Autodesk Inventor part; units mm, degrees
(part 12 of 16)
  spline S72 degree 3 poles (40.8954, 83.9579) (41.0377, 83.8982) (41.1773, 83.832) (41.3128, 83.7584) (41.3531, 83.7365) (41.3931, 83.714) (41.4326, 83.6907) (41.4698, 83.6689) (41.5065, 83.6465) (41.5429, 83.6234) (41.577, 83.6018) (41.6107, 83.5797) (41.644, 83.557) (41.675, 83.5359) (41.7057, 83.5142) (41.7359, 83.4921) (41.764, 83.4715) (41.7917, 83.4506) (41.819, 83.4291) (41.8441, 83.4094) (41.869, 83.3892) (41.8934, 83.3686) (41.9158, 83.3499) (41.9378, 83.3307) (41.9595, 83.3112) (41.9791, 83.2935) (41.9984, 83.2755) (42.0175, 83.2572) (42.0346, 83.2409) (42.0515, 83.2243) (42.0677, 83.2072) (42.082, 83.1922) (42.0958, 83.1767) (42.1105, 83.1616) (42.138, 83.1336) (42.169, 83.1067) (42.1853, 83.0725) (42.1977, 83.0466) (42.2018, 83.0164) (42.2089, 82.9876) (42.2149, 82.9635) (42.223, 82.9404) (42.231, 82.9172) (42.2388, 82.8946) (42.2465, 82.8719) (42.2546, 82.8493) (42.2625, 82.8273) (42.2709, 82.8055) (42.2796, 82.7839) (42.288, 82.7627) (42.2968, 82.7417) (42.3059, 82.7209) (42.3148, 82.7005) (42.324, 82.6804) (42.3336, 82.6603) (42.3429, 82.6408) (42.3526, 82.6215) (42.3626, 82.6023) (42.3724, 82.5836) (42.3824, 82.565) (42.3929, 82.5467) (42.403, 82.5288) (42.4135, 82.511) (42.4244, 82.4935) (42.435, 82.4764) (42.4459, 82.4595) (42.4572, 82.4428) (42.4682, 82.4265) (42.4796, 82.4104) (42.4912, 82.3945) (42.5027, 82.379) (42.5145, 82.3637) (42.5266, 82.3487) (42.5385, 82.3339) (42.5508, 82.3194) (42.5634, 82.3052) (42.5758, 82.2912) (42.5885, 82.2776) (42.6016, 82.2642) (42.6145, 82.251) (42.6278, 82.2382) (42.6414, 82.2257) (42.6548, 82.2133) (42.6687, 82.2012) (42.6828, 82.1896) (42.697, 82.178) (42.7114, 82.1668) (42.7262, 82.1561) (42.7411, 82.1454) (42.7562, 82.1351) (42.7717, 82.1254) (42.7874, 82.1156) (42.8033, 82.1063) (42.8196, 82.0976) (42.8361, 82.0888) (42.853, 82.0806) (42.8701, 82.0731) (42.8876, 82.0654) (42.9055, 82.0584) (42.9236, 82.0522) (42.9421, 82.0459) (42.961, 82.0403) (42.9801, 82.0357) (42.9997, 82.0309) (43.0197, 82.027) (43.0397, 82.0242) (43.0604, 82.0212) (43.0813, 82.0194) (43.1023, 82.0187) (43.1239, 82.0179) (43.1456, 82.0184) (43.1672, 82.0201) (43.1894, 82.0219) (43.2116, 82.025) (43.2335, 82.0295) (43.2559, 82.034) (43.278, 82.04) (43.2996, 82.0472) (43.3151, 82.0524) (43.3303, 82.0581) (43.3454, 82.064) (43.4181, 82.0925) (43.4889, 82.1256) (43.5615, 82.1543) (43.6341, 82.183) (43.7084, 82.2072) (43.7809, 82.2361) (43.796, 82.2421) (43.811, 82.2484) (43.8258, 82.2552) (43.8465, 82.2647) (43.8668, 82.2754) (43.8862, 82.2874) (43.9053, 82.2991) (43.9235, 82.312) (43.941, 82.3259) (43.9579, 82.3394) (43.9741, 82.3539) (43.9894, 82.3692) (44.0041, 82.3841) (44.0181, 82.3997) (44.0313, 82.416) (44.044, 82.4318) (44.0559, 82.4482) (44.0669, 82.4652) (44.0777, 82.4816) (44.0877, 82.4985) (44.0969, 82.5159) (44.1058, 82.5328) (44.1141, 82.55) (44.1216, 82.5676) (44.129, 82.5848) (44.1357, 82.6023) (44.1417, 82.6201) (44.1476, 82.6375) (44.153, 82.6552) (44.1576, 82.6731) (44.1623, 82.6908) (44.1664, 82.7087) (44.1698, 82.7266) (44.1733, 82.7446) (44.1762, 82.7626) (44.1786, 82.7807) (44.181, 82.7989) (44.1829, 82.8171) (44.1843, 82.8354) (44.1857, 82.8538) (44.1865, 82.8722) (44.1869, 82.8907) (44.1874, 82.9094) (44.1873, 82.9281) (44.1868, 82.9467) (44.1863, 82.9657) (44.1853, 82.9847) (44.1839, 83.0036) (44.1825, 83.0228) (44.1807, 83.0421) (44.1784, 83.0612) (44.1761, 83.0808) (44.1734, 83.1003) (44.1703, 83.1198) (44.1671, 83.1396) (44.1635, 83.1595) (44.1595, 83.1792) (44.1555, 83.1994) (44.151, 83.2195) (44.1462, 83.2395) (44.1413, 83.2601) (44.1359, 83.2805) (44.1303, 83.3008) (44.1245, 83.3217) (44.1183, 83.3424) (44.1117, 83.363) (44.105, 83.3842) (44.098, 83.4052) (44.0906, 83.4261) (44.083, 83.4476) (44.075, 83.4689) (44.0668, 83.4901) (44.0583, 83.5119) (44.0495, 83.5335) (44.0402, 83.555) (44.0308, 83.577) (44.0208, 83.5988) (44.011, 83.6206) (44.001, 83.643) (43.9911, 83.6654) (43.979, 83.6871) (43.9646, 83.713) (43.9469, 83.7378) (43.9382, 83.7652) (43.9267, 83.8014) (43.931, 83.8421) (43.9318, 83.8814) (43.9323, 83.9025) (43.9318, 83.9231) (43.9319, 83.9439) (43.9321, 83.9675) (43.9331, 83.9911) (43.9344, 84.0148) (43.9359, 84.0411) (43.9376, 84.0675) (43.9399, 84.0938) (43.9423, 84.1229) (43.9453, 84.1519) (43.9488, 84.1809) (43.9526, 84.2126) (43.957, 84.2443) (43.9618, 84.2759) (43.9671, 84.3102) (43.973, 84.3445) (43.9794, 84.3786) (43.9863, 84.4155) (43.9939, 84.4523) (44.0021, 84.4889) (44.0109, 84.5282) (44.0203, 84.5674) (44.0305, 84.6064) (44.0412, 84.6481) (44.0528, 84.6897) (44.065, 84.731) (44.0779, 84.775) (44.0917, 84.8187) (44.1061, 84.8623) (44.1547, 85.0087) (44.2114, 85.1524) (44.2745, 85.2932) knots 0 0 0 0 0.065113 0.065113 0.065113 0.084473 0.084473 0.084473 0.102659 0.102659 0.102659 0.119672 0.119672 0.119672 0.135512 0.135512 0.135512 0.150178 0.150178 0.150178 0.163672 0.163672 0.163672 0.175991 0.175991 0.175991 0.187138 0.187138 0.187138 0.197111 0.197111 0.197111 0.205911 0.205911 0.205911 0.222284 0.222284 0.222284 0.234681 0.234681 0.234681 0.24506 0.24506 0.24506 0.255176 0.255176 0.255176 0.265035 0.265035 0.265035 0.274643 0.274643 0.274643 0.284008 0.284008 0.284008 0.293139 0.293139 0.293139 0.302047 0.302047 0.302047 0.310743 0.310743 0.310743 0.319241 0.319241 0.319241 0.327556 0.327556 0.327556 0.335706 0.335706 0.335706 0.343713 0.343713 0.343713 0.351599 0.351599 0.351599 0.359392 0.359392 0.359392 0.367126 0.367126 0.367126 0.374835 0.374835 0.374835 0.382562 0.382562 0.382562 0.390352 0.390352 0.390352 0.398256 0.398256 0.398256 0.406325 0.406325 0.406325 0.41461 0.41461 0.41461 0.423156 0.423156 0.423156 0.431994 0.431994 0.431994 0.441132 0.441132 0.441132 0.450548 0.450548 0.450548 0.460189 0.460189 0.460189 0.467051 0.467051 0.467051 0.5 0.5 0.5 0.532949 0.532949 0.532949 0.539811 0.539811 0.539811 0.549452 0.549452 0.549452 0.558868 0.558868 0.558868 0.568006 0.568006 0.568006 0.576844 0.576844 0.576844 0.58539 0.58539 0.58539 0.593675 0.593675 0.593675 0.601744 0.601744 0.601744 0.609648 0.609648 0.609648 0.617438 0.617438 0.617438 0.625165 0.625165 0.625165 0.632874 0.632874 0.632874 0.640608 0.640608 0.640608 0.648401 0.648401 0.648401 0.656287 0.656287 0.656287 0.664294 0.664294 0.664294 0.672444 0.672444 0.672444 0.680759 0.680759 0.680759 0.689257 0.689257 0.689257 0.697953 0.697953 0.697953 0.706861 0.706861 0.706861 0.715992 0.715992 0.715992 0.725357 0.725357 0.725357 0.734965 0.734965 0.734965 0.744824 0.744824 0.744824 0.75494 0.75494 0.75494 0.765319 0.765319 0.765319 0.777716 0.777716 0.777716 0.794089 0.794089 0.794089 0.802889 0.802889 0.802889 0.812862 0.812862 0.812862 0.824009 0.824009 0.824009 0.836328 0.836328 0.836328 0.849822 0.849822 0.849822 0.864488 0.864488 0.864488 0.880328 0.880328 0.880328 0.897341 0.897341 0.897341 0.915527 0.915527 0.915527 0.934887 0.934887 0.934887 1 1 1 1
  arc A275 (40.8954, 83.9579) -> (40.0961, 83.365) centre (45.7832, 76.5321) ccw
  spline S73 degree 3 poles (37.8374, 80.5191) (37.9904, 80.5386) (38.1444, 80.551) (38.2986, 80.5551) (38.3444, 80.5563) (38.3903, 80.5567) (38.4362, 80.5564) (38.4793, 80.556) (38.5223, 80.555) (38.5654, 80.5532) (38.6057, 80.5516) (38.6459, 80.5493) (38.6861, 80.5462) (38.7235, 80.5434) (38.7609, 80.54) (38.7982, 80.536) (38.8327, 80.5322) (38.8672, 80.5279) (38.9016, 80.523) (38.9333, 80.5184) (38.9648, 80.5134) (38.9963, 80.5078) (39.0251, 80.5027) (39.0537, 80.4972) (39.0823, 80.4911) (39.1081, 80.4856) (39.1338, 80.4796) (39.1595, 80.4734) (39.1824, 80.4677) (39.2054, 80.4619) (39.228, 80.4552) (39.2479, 80.4493) (39.2675, 80.4428) (39.2878, 80.4371) (39.3257, 80.4265) (39.3659, 80.4188) (39.3972, 80.3973) (39.4209, 80.3811) (39.4395, 80.3569) (39.4601, 80.3356) (39.4773, 80.3177) (39.4959, 80.3018) (39.5144, 80.2857) (39.5324, 80.27) (39.5504, 80.2541) (39.5687, 80.2386) (39.5866, 80.2236) (39.6047, 80.2089) (39.6231, 80.1945) (39.641, 80.1804) (39.6591, 80.1666) (39.6774, 80.1531) (39.6953, 80.1399) (39.7134, 80.1271) (39.7317, 80.1145) (39.7495, 80.1023) (39.7676, 80.0903) (39.7858, 80.0787) (39.8036, 80.0674) (39.8216, 80.0564) (39.8398, 80.0457) (39.8576, 80.0353) (39.8756, 80.0252) (39.8937, 80.0154) (39.9114, 80.0059) (39.9294, 79.9967) (39.9475, 79.9879) (39.9652, 79.9793) (39.9831, 79.971) (40.0011, 79.9631) (40.0188, 79.9554) (40.0367, 79.948) (40.0547, 79.9411) (40.0724, 79.9343) (40.0902, 79.9278) (40.1082, 79.9219) (40.1259, 79.9159) (40.1438, 79.9105) (40.1618, 79.9054) (40.1796, 79.9005) (40.1975, 79.896) (40.2155, 79.8919) (40.2334, 79.8879) (40.2514, 79.8844) (40.2695, 79.8815) (40.2875, 79.8785) (40.3056, 79.876) (40.3238, 79.8742) (40.342, 79.8723) (40.3603, 79.871) (40.3786, 79.8703) (40.397, 79.8696) (40.4155, 79.8696) (40.4339, 79.8702) (40.4526, 79.8708) (40.4713, 79.8721) (40.49, 79.8742) (40.509, 79.8763) (40.5279, 79.8792) (40.5466, 79.8828) (40.5659, 79.8866) (40.585, 79.8912) (40.6039, 79.8968) (40.6233, 79.9024) (40.6425, 79.9091) (40.6612, 79.9166) (40.6807, 79.9245) (40.6997, 79.9333) (40.7182, 79.9431) (40.7373, 79.9533) (40.7558, 79.9646) (40.7737, 79.9769) (40.7921, 79.9895) (40.8097, 80.0033) (40.8264, 80.0181) (40.8435, 80.0332) (40.8596, 80.0495) (40.8748, 80.0666) (40.8856, 80.0787) (40.8959, 80.0913) (40.9061, 80.104) (40.9548, 80.165) (40.9996, 80.2291) (41.0481, 80.2902) (41.0966, 80.3513) (41.1489, 80.4094) (41.1972, 80.4708) (41.2072, 80.4835) (41.2171, 80.4964) (41.2265, 80.5097) (41.2397, 80.5284) (41.2519, 80.5478) (41.2628, 80.5679) (41.2734, 80.5875) (41.2828, 80.6078) (41.2909, 80.6286) (41.2988, 80.6487) (41.3056, 80.6694) (41.3111, 80.6903) (41.3165, 80.7105) (41.3208, 80.7311) (41.324, 80.7517) (41.3271, 80.7718) (41.3292, 80.7919) (41.3304, 80.8122) (41.3315, 80.8318) (41.3316, 80.8514) (41.3309, 80.871) (41.3303, 80.8901) (41.3288, 80.9092) (41.3265, 80.9282) (41.3243, 80.9468) (41.3213, 80.9653) (41.3177, 80.9837) (41.3141, 81.0018) (41.3098, 81.0198) (41.305, 81.0376) (41.3001, 81.0552) (41.2947, 81.0727) (41.2888, 81.09) (41.2828, 81.1073) (41.2763, 81.1244) (41.2693, 81.1413) (41.2623, 81.1582) (41.2548, 81.1749) (41.2469, 81.1914) (41.2389, 81.2081) (41.2304, 81.2245) (41.2215, 81.2407) (41.2125, 81.2571) (41.2031, 81.2732) (41.1934, 81.2891) (41.1834, 81.3053) (41.1731, 81.3212) (41.1625, 81.3369) (41.1516, 81.3529) (41.1404, 81.3686) (41.1289, 81.3841) (41.1171, 81.3999) (41.105, 81.4154) (41.0925, 81.4307) (41.0798, 81.4463) (41.0668, 81.4617) (41.0535, 81.4768) (41.0399, 81.4923) (41.026, 81.5075) (41.0118, 81.5224) (40.9973, 81.5377) (40.9825, 81.5527) (40.9674, 81.5675) (40.9519, 81.5826) (40.9362, 81.5975) (40.9202, 81.6121) (40.9039, 81.6271) (40.8872, 81.6418) (40.8704, 81.6562) (40.8531, 81.671) (40.8355, 81.6854) (40.8177, 81.6997) (40.7995, 81.7143) (40.7811, 81.7286) (40.7623, 81.7426) (40.7431, 81.7569) (40.7236, 81.7708) (40.7042, 81.7849) (40.6843, 81.7992) (40.6646, 81.8137) (40.6432, 81.8264) (40.6178, 81.8416) (40.5901, 81.8542) (40.5689, 81.8736) (40.5408, 81.8993) (40.5242, 81.9367) (40.5053, 81.9711) (40.4951, 81.9896) (40.4843, 82.0072) (40.4741, 82.0253) (40.4625, 82.0458) (40.4515, 82.0668) (40.4408, 82.0879) (40.4289, 82.1115) (40.4172, 82.1351) (40.406, 82.159) (40.3936, 82.1854) (40.3817, 82.2121) (40.3702, 82.2389) (40.3576, 82.2683) (40.3456, 82.2979) (40.334, 82.3277) (40.3214, 82.3601) (40.3093, 82.3927) (40.2978, 82.4255) (40.2854, 82.4609) (40.2736, 82.4965) (40.2624, 82.5323) (40.2503, 82.5708) (40.2389, 82.6094) (40.2281, 82.6483) (40.2166, 82.6898) (40.2059, 82.7315) (40.1957, 82.7734) (40.185, 82.818) (40.175, 82.8628) (40.1658, 82.9077) (40.1347, 83.0588) (40.1118, 83.2116) (40.0961, 83.365) knots 0 0 0 0 0.065113 0.065113 0.065113 0.084473 0.084473 0.084473 0.102659 0.102659 0.102659 0.119672 0.119672 0.119672 0.135512 0.135512 0.135512 0.150178 0.150178 0.150178 0.163672 0.163672 0.163672 0.175991 0.175991 0.175991 0.187138 0.187138 0.187138 0.197111 0.197111 0.197111 0.205911 0.205911 0.205911 0.222284 0.222284 0.222284 0.234681 0.234681 0.234681 0.24506 0.24506 0.24506 0.255176 0.255176 0.255176 0.265035 0.265035 0.265035 0.274643 0.274643 0.274643 0.284008 0.284008 0.284008 0.293139 0.293139 0.293139 0.302047 0.302047 0.302047 0.310743 0.310743 0.310743 0.319241 0.319241 0.319241 0.327556 0.327556 0.327556 0.335706 0.335706 0.335706 0.343713 0.343713 0.343713 0.351599 0.351599 0.351599 0.359392 0.359392 0.359392 0.367126 0.367126 0.367126 0.374835 0.374835 0.374835 0.382562 0.382562 0.382562 0.390352 0.390352 0.390352 0.398256 0.398256 0.398256 0.406325 0.406325 0.406325 0.41461 0.41461 0.41461 0.423156 0.423156 0.423156 0.431994 0.431994 0.431994 0.441132 0.441132 0.441132 0.450548 0.450548 0.450548 0.460189 0.460189 0.460189 0.467051 0.467051 0.467051 0.5 0.5 0.5 0.532949 0.532949 0.532949 0.539811 0.539811 0.539811 0.549452 0.549452 0.549452 0.558868 0.558868 0.558868 0.568006 0.568006 0.568006 0.576844 0.576844 0.576844 0.58539 0.58539 0.58539 0.593675 0.593675 0.593675 0.601744 0.601744 0.601744 0.609648 0.609648 0.609648 0.617438 0.617438 0.617438 0.625165 0.625165 0.625165 0.632874 0.632874 0.632874 0.640608 0.640608 0.640608 0.648401 0.648401 0.648401 0.656287 0.656287 0.656287 0.664294 0.664294 0.664294 0.672444 0.672444 0.672444 0.680759 0.680759 0.680759 0.689257 0.689257 0.689257 0.697953 0.697953 0.697953 0.706861 0.706861 0.706861 0.715992 0.715992 0.715992 0.725357 0.725357 0.725357 0.734965 0.734965 0.734965 0.744824 0.744824 0.744824 0.75494 0.75494 0.75494 0.765319 0.765319 0.765319 0.777716 0.777716 0.777716 0.794089 0.794089 0.794089 0.802889 0.802889 0.802889 0.812862 0.812862 0.812862 0.824009 0.824009 0.824009 0.836328 0.836328 0.836328 0.849822 0.849822 0.849822 0.864488 0.864488 0.864488 0.880328 0.880328 0.880328 0.897341 0.897341 0.897341 0.915527 0.915527 0.915527 0.934887 0.934887 0.934887 1 1 1 1
  arc A276 (37.8374, 80.5191) -> (37.4416, 79.606) centre (45.7832, 76.5321) ccw
  spline S74 degree 3 poles (36.9084, 76.012) (37.0312, 76.1054) (37.1584, 76.1932) (37.2899, 76.2738) (37.329, 76.2977) (37.3685, 76.3211) (37.4084, 76.3437) (37.4459, 76.365) (37.4837, 76.3856) (37.5219, 76.4056) (37.5576, 76.4243) (37.5936, 76.4424) (37.6299, 76.4599) (37.6637, 76.4762) (37.6978, 76.4919) (37.7321, 76.507) (37.7639, 76.5211) (37.7959, 76.5346) (37.8282, 76.5475) (37.8578, 76.5594) (37.8877, 76.5708) (37.9177, 76.5817) (37.9452, 76.5917) (37.9728, 76.6012) (38.0005, 76.6102) (38.0256, 76.6184) (38.0509, 76.6261) (38.0763, 76.6335) (38.099, 76.6401) (38.1218, 76.6465) (38.1447, 76.652) (38.1649, 76.6568) (38.1851, 76.661) (38.2056, 76.6663) (38.2436, 76.676) (38.2823, 76.6894) (38.3202, 76.6865) (38.3488, 76.6842) (38.377, 76.6727) (38.4055, 76.6645) (38.4293, 76.6576) (38.4534, 76.6531) (38.4775, 76.6484) (38.501, 76.6438) (38.5245, 76.6391) (38.5481, 76.6348) (38.5711, 76.6307) (38.5941, 76.6271) (38.6173, 76.6237) (38.6398, 76.6205) (38.6624, 76.6176) (38.685, 76.6151) (38.707, 76.6126) (38.7291, 76.6105) (38.7512, 76.6088) (38.7728, 76.6071) (38.7944, 76.6058) (38.816, 76.6049) (38.8371, 76.604) (38.8582, 76.6034) (38.8793, 76.6033) (38.8999, 76.6031) (38.9205, 76.6034) (38.9411, 76.604) (38.9612, 76.6046) (38.9813, 76.6056) (39.0014, 76.607) (39.0211, 76.6084) (39.0407, 76.6102) (39.0603, 76.6124) (39.0795, 76.6146) (39.0986, 76.6171) (39.1177, 76.6201) (39.1364, 76.6231) (39.1551, 76.6264) (39.1737, 76.6302) (39.192, 76.634) (39.2102, 76.6382) (39.2283, 76.6428) (39.2462, 76.6474) (39.2639, 76.6524) (39.2816, 76.658) (39.299, 76.6634) (39.3164, 76.6694) (39.3335, 76.6759) (39.3506, 76.6823) (39.3675, 76.6892) (39.3842, 76.6967) (39.4009, 76.7042) (39.4174, 76.7122) (39.4336, 76.7207) (39.4499, 76.7294) (39.4659, 76.7386) (39.4816, 76.7483) (39.4975, 76.7582) (39.513, 76.7687) (39.5281, 76.7798) (39.5435, 76.7911) (39.5585, 76.8031) (39.5729, 76.8156) (39.5877, 76.8285) (39.6019, 76.8421) (39.6155, 76.8563) (39.6294, 76.8709) (39.6427, 76.8863) (39.6552, 76.9022) (39.6681, 76.9187) (39.6802, 76.9359) (39.6913, 76.9536) (39.7027, 76.972) (39.7132, 76.991) (39.7225, 77.0106) (39.7321, 77.0307) (39.7405, 77.0515) (39.7475, 77.0726) (39.7548, 77.0943) (39.7606, 77.1165) (39.7652, 77.1388) (39.7685, 77.1548) (39.7711, 77.1708) (39.7736, 77.1869) (39.7853, 77.2641) (39.792, 77.342) (39.8034, 77.4191) (39.8149, 77.4963) (39.8311, 77.5728) (39.8423, 77.6501) (39.8446, 77.6661) (39.8467, 77.6823) (39.8482, 77.6985) (39.8503, 77.7212) (39.8512, 77.7441) (39.8505, 77.7669) (39.8499, 77.7893) (39.8479, 77.8115) (39.8445, 77.8336) (39.8413, 77.855) (39.8369, 77.8762) (39.8312, 77.8972) (39.8258, 77.9174) (39.8192, 77.9373) (39.8117, 77.9568) (39.8043, 77.9757) (39.7961, 77.9942) (39.7869, 78.0123) (39.7781, 78.0298) (39.7684, 78.0469) (39.758, 78.0636) (39.7478, 78.0798) (39.737, 78.0956) (39.7255, 78.1109) (39.7143, 78.1259) (39.7025, 78.1404) (39.6902, 78.1545) (39.678, 78.1684) (39.6653, 78.1818) (39.6522, 78.1948) (39.6392, 78.2077) (39.6258, 78.2202) (39.612, 78.2322) (39.5982, 78.2441) (39.584, 78.2557) (39.5695, 78.2668) (39.555, 78.278) (39.5401, 78.2887) (39.525, 78.299) (39.5097, 78.3094) (39.4942, 78.3194) (39.4784, 78.329) (39.4624, 78.3387) (39.4462, 78.348) (39.4298, 78.3569) (39.4131, 78.3659) (39.3962, 78.3746) (39.3791, 78.3828) (39.3618, 78.3912) (39.3442, 78.3992) (39.3265, 78.4069) (39.3084, 78.4147) (39.2901, 78.4221) (39.2717, 78.4291) (39.2529, 78.4363) (39.2339, 78.4431) (39.2149, 78.4495) (39.1953, 78.4561) (39.1757, 78.4623) (39.1559, 78.4681) (39.1357, 78.4741) (39.1153, 78.4797) (39.0949, 78.485) (39.074, 78.4904) (39.0529, 78.4954) (39.0318, 78.5) (39.0101, 78.5048) (38.9884, 78.5092) (38.9665, 78.5133) (38.9442, 78.5174) (38.9217, 78.5212) (38.8992, 78.5246) (38.8761, 78.5282) (38.853, 78.5314) (38.8298, 78.5341) (38.806, 78.5369) (38.7821, 78.5392) (38.7583, 78.5416) (38.7339, 78.5441) (38.7095, 78.5468) (38.6847, 78.5471) (38.6551, 78.5475) (38.6248, 78.5446) (38.5967, 78.5508) (38.5596, 78.559) (38.5265, 78.5831) (38.4929, 78.6034) (38.4749, 78.6144) (38.4567, 78.6243) (38.4388, 78.6348) (38.4185, 78.6467) (38.3985, 78.6594) (38.3787, 78.6724) (38.3566, 78.6868) (38.3346, 78.7015) (38.313, 78.7166) (38.289, 78.7332) (38.2654, 78.7504) (38.242, 78.7679) (38.2164, 78.787) (38.1912, 78.8066) (38.1662, 78.8266) (38.1391, 78.8484) (38.1124, 78.8706) (38.0861, 78.8932) (38.0576, 78.9177) (38.0295, 78.9426) (38.0019, 78.968) (37.9722, 78.9953) (37.943, 79.0231) (37.9143, 79.0513) (37.8836, 79.0815) (37.8534, 79.1123) (37.8237, 79.1435) (37.7921, 79.1767) (37.7611, 79.2105) (37.7306, 79.2448) (37.6281, 79.3601) (37.532, 79.481) (37.4416, 79.606) knots 0 0 0 0 0.065113 0.065113 0.065113 0.084473 0.084473 0.084473 0.102659 0.102659 0.102659 0.119672 0.119672 0.119672 0.135512 0.135512 0.135512 0.150178 0.150178 0.150178 0.163672 0.163672 0.163672 0.175991 0.175991 0.175991 0.187138 0.187138 0.187138 0.197111 0.197111 0.197111 0.205911 0.205911 0.205911 0.222284 0.222284 0.222284 0.234681 0.234681 0.234681 0.24506 0.24506 0.24506 0.255176 0.255176 0.255176 0.265035 0.265035 0.265035 0.274643 0.274643 0.274643 0.284008 0.284008 0.284008 0.293139 0.293139 0.293139 0.302047 0.302047 0.302047 0.310743 0.310743 0.310743 0.319241 0.319241 0.319241 0.327556 0.327556 0.327556 0.335706 0.335706 0.335706 0.343713 0.343713 0.343713 0.351599 0.351599 0.351599 0.359392 0.359392 0.359392 0.367126 0.367126 0.367126 0.374835 0.374835 0.374835 0.382562 0.382562 0.382562 0.390352 0.390352 0.390352 0.398256 0.398256 0.398256 0.406325 0.406325 0.406325 0.41461 0.41461 0.41461 0.423156 0.423156 0.423156 0.431994 0.431994 0.431994 0.441132 0.441132 0.441132 0.450548 0.450548 0.450548 0.460189 0.460189 0.460189 0.467051 0.467051 0.467051 0.5 0.5 0.5 0.532949 0.532949 0.532949 0.539811 0.539811 0.539811 0.549452 0.549452 0.549452 0.558868 0.558868 0.558868 0.568006 0.568006 0.568006 0.576844 0.576844 0.576844 0.58539 0.58539 0.58539 0.593675 0.593675 0.593675 0.601744 0.601744 0.601744 0.609648 0.609648 0.609648 0.617438 0.617438 0.617438 0.625165 0.625165 0.625165 0.632874 0.632874 0.632874 0.640608 0.640608 0.640608 0.648401 0.648401 0.648401 0.656287 0.656287 0.656287 0.664294 0.664294 0.664294 0.672444 0.672444 0.672444 0.680759 0.680759 0.680759 0.689257 0.689257 0.689257 0.697953 0.697953 0.697953 0.706861 0.706861 0.706861 0.715992 0.715992 0.715992 0.725357 0.725357 0.725357 0.734965 0.734965 0.734965 0.744824 0.744824 0.744824 0.75494 0.75494 0.75494 0.765319 0.765319 0.765319 0.777716 0.777716 0.777716 0.794089 0.794089 0.794089 0.802889 0.802889 0.802889 0.812862 0.812862 0.812862 0.824009 0.824009 0.824009 0.836328 0.836328 0.836328 0.849822 0.849822 0.849822 0.864488 0.864488 0.864488 0.880328 0.880328 0.880328 0.897341 0.897341 0.897341 0.915527 0.915527 0.915527 0.934887 0.934887 0.934887 1 1 1 1
  arc A277 (36.9084, 76.012) -> (37.0222, 75.0234) centre (45.7832, 76.5321) ccw
  spline S75 degree 3 poles (38.3575, 71.6443) (38.4171, 71.7866) (38.4833, 71.9262) (38.557, 72.0617) (38.5788, 72.102) (38.6014, 72.142) (38.6246, 72.1815) (38.6465, 72.2187) (38.6689, 72.2555) (38.6919, 72.2919) (38.7135, 72.3259) (38.7356, 72.3596) (38.7583, 72.3929) (38.7795, 72.4239) (38.8011, 72.4546) (38.8233, 72.4849) (38.8438, 72.5129) (38.8648, 72.5406) (38.8863, 72.5679) (38.906, 72.5931) (38.9262, 72.6179) (38.9467, 72.6423) (38.9655, 72.6647) (38.9846, 72.6867) (39.0042, 72.7084) (39.0219, 72.728) (39.0399, 72.7473) (39.0581, 72.7664) (39.0745, 72.7835) (39.0911, 72.8004) (39.1081, 72.8166) (39.1232, 72.831) (39.1386, 72.8447) (39.1537, 72.8595) (39.1818, 72.8869) (39.2086, 72.9179) (39.2429, 72.9343) (39.2688, 72.9467) (39.299, 72.9507) (39.3278, 72.9579) (39.3518, 72.9638) (39.3749, 72.972) (39.3981, 72.9799) (39.4208, 72.9877) (39.4435, 72.9954) (39.4661, 73.0035) (39.488, 73.0114) (39.5098, 73.0198) (39.5315, 73.0285) (39.5526, 73.037) (39.5737, 73.0457) (39.5945, 73.0548) (39.6148, 73.0637) (39.635, 73.073) (39.655, 73.0825) (39.6745, 73.0919) (39.6939, 73.1015) (39.7131, 73.1115) (39.7318, 73.1213) (39.7503, 73.1314) (39.7687, 73.1418) (39.7866, 73.152) (39.8043, 73.1625) (39.8218, 73.1733) (39.839, 73.1839) (39.8559, 73.1948) (39.8726, 73.2061) (39.8889, 73.2171) (39.905, 73.2285) (39.9208, 73.2402) (39.9364, 73.2516) (39.9517, 73.2634) (39.9667, 73.2756) (39.9815, 73.2875) (39.996, 73.2997) (40.0101, 73.3123) (40.0241, 73.3247) (40.0378, 73.3374) (40.0512, 73.3505) (40.0643, 73.3634) (40.0772, 73.3767) (40.0897, 73.3903) (40.1021, 73.4038) (40.1141, 73.4176) (40.1258, 73.4318) (40.1373, 73.4459) (40.1485, 73.4603) (40.1592, 73.4751) (40.17, 73.49) (40.1802, 73.5052) (40.19, 73.5207) (40.1998, 73.5363) (40.2091, 73.5522) (40.2178, 73.5685) (40.2266, 73.5851) (40.2348, 73.6019) (40.2423, 73.6191) (40.25, 73.6366) (40.257, 73.6544) (40.2631, 73.6725) (40.2695, 73.6911) (40.275, 73.7099) (40.2797, 73.729) (40.2845, 73.7487) (40.2883, 73.7686) (40.2912, 73.7886) (40.2941, 73.8094) (40.296, 73.8303) (40.2967, 73.8512) (40.2974, 73.8728) (40.2969, 73.8945) (40.2952, 73.9161) (40.2935, 73.9384) (40.2904, 73.9605) (40.2859, 73.9824) (40.2813, 74.0048) (40.2753, 74.0269) (40.2681, 74.0486) (40.263, 74.064) (40.2573, 74.0792) (40.2513, 74.0943) (40.2229, 74.167) (40.1898, 74.2379) (40.1611, 74.3104) (40.1324, 74.383) (40.1082, 74.4573) (40.0793, 74.5298) (40.0732, 74.5449) (40.067, 74.5599) (40.0602, 74.5747) (40.0506, 74.5955) (40.0399, 74.6157) (40.028, 74.6352) (40.0163, 74.6542) (40.0034, 74.6724) (39.9894, 74.6899) (39.9759, 74.7068) (39.9615, 74.723) (39.9461, 74.7383) (39.9313, 74.7531) (39.9157, 74.7671) (39.8993, 74.7802) (39.8836, 74.7929) (39.8671, 74.8048) (39.8502, 74.8159) (39.8338, 74.8266) (39.8168, 74.8366) (39.7995, 74.8458) (39.7826, 74.8548) (39.7653, 74.863) (39.7478, 74.8705) (39.7305, 74.8779) (39.713, 74.8846) (39.6953, 74.8906) (39.6778, 74.8966) (39.6601, 74.9019) (39.6423, 74.9066) (39.6246, 74.9112) (39.6067, 74.9153) (39.5887, 74.9188) (39.5708, 74.9223) (39.5528, 74.9252) (39.5347, 74.9276) (39.5165, 74.93) (39.4983, 74.9318) (39.48, 74.9332) (39.4616, 74.9346) (39.4431, 74.9355) (39.4247, 74.9359) (39.406, 74.9363) (39.3873, 74.9362) (39.3686, 74.9357) (39.3497, 74.9352) (39.3307, 74.9342) (39.3118, 74.9328) (39.2925, 74.9314) (39.2733, 74.9296) (39.2541, 74.9273) (39.2346, 74.925) (39.2151, 74.9223) (39.1956, 74.9192) (39.1757, 74.916) (39.1559, 74.9124) (39.1362, 74.9084) (39.116, 74.9044) (39.0959, 74.8999) (39.0758, 74.8951) (39.0553, 74.8902) (39.0349, 74.8849) (39.0145, 74.8792) (38.9937, 74.8734) (38.973, 74.8672) (38.9524, 74.8607) (38.9312, 74.854) (38.9102, 74.8469) (38.8893, 74.8395) (38.8678, 74.8319) (38.8465, 74.8239) (38.8253, 74.8157) (38.8035, 74.8072) (38.7819, 74.7984) (38.7604, 74.7892) (38.7384, 74.7797) (38.7166, 74.7697) (38.6947, 74.7599) (38.6723, 74.7499) (38.6499, 74.74) (38.6283, 74.7279) (38.6024, 74.7135) (38.5776, 74.6958) (38.5502, 74.6871) (38.514, 74.6757) (38.4732, 74.6799) (38.434, 74.6808) (38.4129, 74.6812) (38.3922, 74.6807) (38.3714, 74.6809) (38.3479, 74.681) (38.3242, 74.6821) (38.3006, 74.6834) (38.2742, 74.6848) (38.2479, 74.6866) (38.2216, 74.6888) (38.1925, 74.6913) (38.1635, 74.6943) (38.1345, 74.6977) (38.1027, 74.7015) (38.0711, 74.7059) (38.0395, 74.7107) (38.0051, 74.716) (37.9709, 74.7219) (37.9367, 74.7283) (37.8999, 74.7353) (37.8631, 74.7428) (37.8265, 74.751) (37.7871, 74.7598) (37.748, 74.7693) (37.7089, 74.7794) (37.6672, 74.7902) (37.6257, 74.8017) (37.5844, 74.8139) (37.5404, 74.8269) (37.4966, 74.8406) (37.4531, 74.8551) (37.3067, 74.9037) (37.163, 74.9603) (37.0222, 75.0234) knots 0 0 0 0 0.065113 0.065113 0.065113 0.084473 0.084473 0.084473 0.102659 0.102659 0.102659 0.119672 0.119672 0.119672 0.135512 0.135512 0.135512 0.150178 0.150178 0.150178 0.163672 0.163672 0.163672 0.175991 0.175991 0.175991 0.187138 0.187138 0.187138 0.197111 0.197111 0.197111 0.205911 0.205911 0.205911 0.222284 0.222284 0.222284 0.234681 0.234681 0.234681 0.24506 0.24506 0.24506 0.255176 0.255176 0.255176 0.265035 0.265035 0.265035 0.274643 0.274643 0.274643 0.284008 0.284008 0.284008 0.293139 0.293139 0.293139 0.302047 0.302047 0.302047 0.310743 0.310743 0.310743 0.319241 0.319241 0.319241 0.327556 0.327556 0.327556 0.335706 0.335706 0.335706 0.343713 0.343713 0.343713 0.351599 0.351599 0.351599 0.359392 0.359392 0.359392 0.367126 0.367126 0.367126 0.374835 0.374835 0.374835 0.382562 0.382562 0.382562 0.390352 0.390352 0.390352 0.398256 0.398256 0.398256 0.406325 0.406325 0.406325 0.41461 0.41461 0.41461 0.423156 0.423156 0.423156 0.431994 0.431994 0.431994 0.441132 0.441132 0.441132 0.450548 0.450548 0.450548 0.460189 0.460189 0.460189 0.467051 0.467051 0.467051 0.5 0.5 0.5 0.532949 0.532949 0.532949 0.539811 0.539811 0.539811 0.549452 0.549452 0.549452 0.558868 0.558868 0.558868 0.568006 0.568006 0.568006 0.576844 0.576844 0.576844 0.58539 0.58539 0.58539 0.593675 0.593675 0.593675 0.601744 0.601744 0.601744 0.609648 0.609648 0.609648 0.617438 0.617438 0.617438 0.625165 0.625165 0.625165 0.632874 0.632874 0.632874 0.640608 0.640608 0.640608 0.648401 0.648401 0.648401 0.656287 0.656287 0.656287 0.664294 0.664294 0.664294 0.672444 0.672444 0.672444 0.680759 0.680759 0.680759 0.689257 0.689257 0.689257 0.697953 0.697953 0.697953 0.706861 0.706861 0.706861 0.715992 0.715992 0.715992 0.725357 0.725357 0.725357 0.734965 0.734965 0.734965 0.744824 0.744824 0.744824 0.75494 0.75494 0.75494 0.765319 0.765319 0.765319 0.777716 0.777716 0.777716 0.794089 0.794089 0.794089 0.802889 0.802889 0.802889 0.812862 0.812862 0.812862 0.824009 0.824009 0.824009 0.836328 0.836328 0.836328 0.849822 0.849822 0.849822 0.864488 0.864488 0.864488 0.880328 0.880328 0.880328 0.897341 0.897341 0.897341 0.915527 0.915527 0.915527 0.934887 0.934887 0.934887 1 1 1 1
  arc A278 (38.3575, 71.6443) -> (38.9503, 70.845) centre (45.7832, 76.5321) ccw
  spline S76 degree 3 poles (41.7963, 68.5863) (41.7768, 68.7393) (41.7643, 68.8933) (41.7603, 69.0475) (41.7591, 69.0934) (41.7587, 69.1392) (41.759, 69.1851) (41.7593, 69.2282) (41.7604, 69.2713) (41.7621, 69.3143) (41.7638, 69.3546) (41.7661, 69.3948) (41.7691, 69.435) (41.7719, 69.4724) (41.7753, 69.5098) (41.7794, 69.5471) (41.7832, 69.5817) (41.7875, 69.6161) (41.7924, 69.6505) (41.7969, 69.6822) (41.802, 69.7138) (41.8075, 69.7452) (41.8126, 69.774) (41.8182, 69.8026) (41.8243, 69.8312) (41.8298, 69.857) (41.8357, 69.8827) (41.842, 69.9084) (41.8476, 69.9314) (41.8535, 69.9543) (41.8602, 69.9769) (41.8661, 69.9968) (41.8726, 70.0164) (41.8782, 70.0368) (41.8888, 70.0746) (41.8966, 70.1148) (41.9181, 70.1461) (41.9343, 70.1698) (41.9584, 70.1884) (41.9798, 70.209) (41.9976, 70.2262) (42.0136, 70.2448) (42.0297, 70.2633) (42.0454, 70.2814) (42.0612, 70.2994) (42.0767, 70.3177) (42.0918, 70.3355) (42.1065, 70.3537) (42.1209, 70.372) (42.135, 70.3899) (42.1488, 70.408) (42.1623, 70.4264) (42.1754, 70.4442) (42.1883, 70.4623) (42.2009, 70.4806) (42.2131, 70.4984) (42.225, 70.5165) (42.2366, 70.5347) (42.248, 70.5525) (42.259, 70.5705) (42.2697, 70.5887) (42.2801, 70.6065) (42.2902, 70.6245) (42.2999, 70.6426) (42.3095, 70.6604) (42.3186, 70.6783) (42.3275, 70.6964) (42.3361, 70.7141) (42.3444, 70.732) (42.3522, 70.75) (42.36, 70.7677) (42.3673, 70.7856) (42.3743, 70.8036) (42.3811, 70.8213) (42.3875, 70.8391) (42.3935, 70.8571) (42.3994, 70.8749) (42.4049, 70.8927) (42.4099, 70.9107) (42.4149, 70.9285) (42.4194, 70.9464) (42.4234, 70.9645) (42.4274, 70.9823) (42.4309, 71.0003) (42.4339, 71.0184) (42.4369, 71.0364) (42.4393, 71.0545) (42.4412, 71.0727) (42.4431, 71.0909) (42.4444, 71.1092) (42.4451, 71.1275) (42.4457, 71.1459) (42.4458, 71.1644) (42.4452, 71.1828) (42.4446, 71.2016) (42.4432, 71.2203) (42.4412, 71.2389) (42.4391, 71.2579) (42.4362, 71.2768) (42.4325, 71.2956) (42.4288, 71.3148) (42.4241, 71.3339) (42.4186, 71.3528) (42.4129, 71.3722) (42.4063, 71.3914) (42.3987, 71.4102) (42.3909, 71.4296) (42.3821, 71.4486) (42.3722, 71.4671) (42.362, 71.4862) (42.3508, 71.5048) (42.3385, 71.5226) (42.3258, 71.541) (42.3121, 71.5586) (42.2973, 71.5753) (42.2821, 71.5924) (42.2659, 71.6086) (42.2488, 71.6237) (42.2366, 71.6345) (42.2241, 71.6449) (42.2114, 71.655) (42.1504, 71.7037) (42.0863, 71.7485) (42.0252, 71.797) (41.9641, 71.8455) (41.9059, 71.8978) (41.8446, 71.9461) (41.8318, 71.9562) (41.8189, 71.9661) (41.8057, 71.9754) (41.787, 71.9886) (41.7676, 72.0008) (41.7475, 72.0117) (41.7279, 72.0223) (41.7076, 72.0317) (41.6868, 72.0398) (41.6666, 72.0477) (41.646, 72.0545) (41.6251, 72.0601) (41.6048, 72.0655) (41.5843, 72.0698) (41.5636, 72.073) (41.5436, 72.0761) (41.5234, 72.0782) (41.5032, 72.0793) (41.4836, 72.0804) (41.464, 72.0805) (41.4443, 72.0799) (41.4252, 72.0792) (41.4061, 72.0777) (41.3872, 72.0754) (41.3686, 72.0732) (41.3501, 72.0702) (41.3317, 72.0666) (41.3136, 72.063) (41.2956, 72.0587) (41.2778, 72.0539) (41.2601, 72.0491) (41.2426, 72.0436) (41.2253, 72.0377) (41.2081, 72.0317) (41.191, 72.0252) (41.1741, 72.0183) (41.1572, 72.0112) (41.1404, 72.0037) (41.1239, 71.9958) (41.1073, 71.9878) (41.0909, 71.9793) (41.0747, 71.9704) (41.0583, 71.9615) (41.0421, 71.9521) (41.0262, 71.9423) (41.0101, 71.9324) (40.9941, 71.9221) (40.9784, 71.9114) (40.9625, 71.9005) (40.9468, 71.8893) (40.9313, 71.8778) (40.9155, 71.866) (40.8999, 71.8539) (40.8847, 71.8415) (40.869, 71.8288) (40.8537, 71.8158) (40.8386, 71.8025) (40.8231, 71.7888) (40.8079, 71.7749) (40.793, 71.7607) (40.7777, 71.7462) (40.7626, 71.7314) (40.7479, 71.7163) (40.7327, 71.7009) (40.7179, 71.6851) (40.7033, 71.6692) (40.6883, 71.6528) (40.6736, 71.6362) (40.6592, 71.6193) (40.6444, 71.602) (40.6299, 71.5844) (40.6157, 71.5667) (40.6011, 71.5484) (40.5867, 71.53) (40.5728, 71.5113) (40.5585, 71.492) (40.5445, 71.4725) (40.5305, 71.4531) (40.5161, 71.4332) (40.5017, 71.4135) (40.4889, 71.3922) (40.4738, 71.3667) (40.4611, 71.339) (40.4417, 71.3178) (40.4161, 71.2898) (40.3787, 71.2731) (40.3443, 71.2542) (40.3258, 71.244) (40.3081, 71.2333) (40.2901, 71.223) (40.2696, 71.2114) (40.2486, 71.2004) (40.2275, 71.1897) (40.2039, 71.1778) (40.1802, 71.1662) (40.1563, 71.1549) (40.1299, 71.1425) (40.1033, 71.1306) (40.0764, 71.1191) (40.047, 71.1066) (40.0174, 71.0945) (39.9876, 71.0829) (39.9553, 71.0703) (39.9227, 71.0582) (39.8899, 71.0467) (39.8545, 71.0343) (39.8188, 71.0225) (39.783, 71.0113) (39.7446, 70.9992) (39.7059, 70.9878) (39.6671, 70.9771) (39.6256, 70.9656) (39.5838, 70.9548) (39.5419, 70.9447) (39.4974, 70.9339) (39.4526, 70.9239) (39.4077, 70.9147) (39.2566, 70.8836) (39.1038, 70.8608) (38.9503, 70.845) knots 0 0 0 0 0.065113 0.065113 0.065113 0.084473 0.084473 0.084473 0.102659 0.102659 0.102659 0.119672 0.119672 0.119672 0.135512 0.135512 0.135512 0.150178 0.150178 0.150178 0.163672 0.163672 0.163672 0.175991 0.175991 0.175991 0.187138 0.187138 0.187138 0.197111 0.197111 0.197111 0.205911 0.205911 0.205911 0.222284 0.222284 0.222284 0.234681 0.234681 0.234681 0.24506 0.24506 0.24506 0.255176 0.255176 0.255176 0.265035 0.265035 0.265035 0.274643 0.274643 0.274643 0.284008 0.284008 0.284008 0.293139 0.293139 0.293139 0.302047 0.302047 0.302047 0.310743 0.310743 0.310743 0.319241 0.319241 0.319241 0.327556 0.327556 0.327556 0.335706 0.335706 0.335706 0.343713 0.343713 0.343713 0.351599 0.351599 0.351599 0.359392 0.359392 0.359392 0.367126 0.367126 0.367126 0.374835 0.374835 0.374835 0.382562 0.382562 0.382562 0.390352 0.390352 0.390352 0.398256 0.398256 0.398256 0.406325 0.406325 0.406325 0.41461 0.41461 0.41461 0.423156 0.423156 0.423156 0.431994 0.431994 0.431994 0.441132 0.441132 0.441132 0.450548 0.450548 0.450548 0.460189 0.460189 0.460189 0.467051 0.467051 0.467051 0.5 0.5 0.5 0.532949 0.532949 0.532949 0.539811 0.539811 0.539811 0.549452 0.549452 0.549452 0.558868 0.558868 0.558868 0.568006 0.568006 0.568006 0.576844 0.576844 0.576844 0.58539 0.58539 0.58539 0.593675 0.593675 0.593675 0.601744 0.601744 0.601744 0.609648 0.609648 0.609648 0.617438 0.617438 0.617438 0.625165 0.625165 0.625165 0.632874 0.632874 0.632874 0.640608 0.640608 0.640608 0.648401 0.648401 0.648401 0.656287 0.656287 0.656287 0.664294 0.664294 0.664294 0.672444 0.672444 0.672444 0.680759 0.680759 0.680759 0.689257 0.689257 0.689257 0.697953 0.697953 0.697953 0.706861 0.706861 0.706861 0.715992 0.715992 0.715992 0.725357 0.725357 0.725357 0.734965 0.734965 0.734965 0.744824 0.744824 0.744824 0.75494 0.75494 0.75494 0.765319 0.765319 0.765319 0.777716 0.777716 0.777716 0.794089 0.794089 0.794089 0.802889 0.802889 0.802889 0.812862 0.812862 0.812862 0.824009 0.824009 0.824009 0.836328 0.836328 0.836328 0.849822 0.849822 0.849822 0.864488 0.864488 0.864488 0.880328 0.880328 0.880328 0.897341 0.897341 0.897341 0.915527 0.915527 0.915527 0.934887 0.934887 0.934887 1 1 1 1
  arc A279 (41.7963, 68.5863) -> (42.7093, 68.1905) centre (45.7832, 76.5321) ccw
  spline S77 degree 3 poles (46.3033, 67.6574) (46.2099, 67.7802) (46.1222, 67.9073) (46.0416, 68.0388) (46.0176, 68.0779) (45.9943, 68.1174) (45.9717, 68.1573) (45.9504, 68.1948) (45.9298, 68.2326) (45.9098, 68.2708) (45.8911, 68.3065) (45.873, 68.3425) (45.8555, 68.3788) (45.8392, 68.4126) (45.8235, 68.4467) (45.8083, 68.481) (45.7943, 68.5128) (45.7808, 68.5448) (45.7679, 68.5771) (45.756, 68.6068) (45.7445, 68.6366) (45.7336, 68.6667) (45.7237, 68.6941) (45.7141, 68.7217) (45.7051, 68.7495) (45.697, 68.7746) (45.6893, 68.7998) (45.6819, 68.8252) (45.6753, 68.8479) (45.6689, 68.8707) (45.6634, 68.8936) (45.6585, 68.9138) (45.6543, 68.9341) (45.6491, 68.9545) (45.6393, 68.9925) (45.626, 69.0312) (45.6289, 69.0691) (45.6311, 69.0978) (45.6427, 69.1259) (45.6509, 69.1544) (45.6578, 69.1782) (45.6623, 69.2023) (45.667, 69.2264) (45.6715, 69.2499) (45.6763, 69.2734) (45.6805, 69.297) (45.6847, 69.32) (45.6883, 69.3431) (45.6916, 69.3662) (45.6949, 69.3887) (45.6978, 69.4113) (45.7003, 69.4339) (45.7028, 69.456) (45.7049, 69.478) (45.7066, 69.5002) (45.7083, 69.5217) (45.7096, 69.5433) (45.7105, 69.5649) (45.7114, 69.586) (45.7119, 69.6071) (45.7121, 69.6282) (45.7122, 69.6488) (45.712, 69.6694) (45.7114, 69.69) (45.7107, 69.7102) (45.7097, 69.7303) (45.7083, 69.7503) (45.7069, 69.77) (45.7052, 69.7896) (45.703, 69.8092) (45.7008, 69.8284) (45.6982, 69.8475) (45.6953, 69.8666) (45.6923, 69.8853) (45.689, 69.904) (45.6851, 69.9226) (45.6814, 69.9409) (45.6772, 69.9591) (45.6726, 69.9772) (45.668, 69.9951) (45.6629, 70.0129) (45.6574, 70.0305) (45.6519, 70.048) (45.646, 70.0653) (45.6395, 70.0824) (45.6331, 70.0995) (45.6261, 70.1164) (45.6187, 70.1331) (45.6112, 70.1498) (45.6032, 70.1663) (45.5946, 70.1825) (45.586, 70.1988) (45.5768, 70.2148) (45.5671, 70.2305) (45.5572, 70.2464) (45.5467, 70.2619) (45.5356, 70.277) (45.5242, 70.2924) (45.5123, 70.3074) (45.4997, 70.3218) (45.4868, 70.3366) (45.4733, 70.3508) (45.4591, 70.3644) (45.4444, 70.3784) (45.4291, 70.3917) (45.4132, 70.4041) (45.3967, 70.4171) (45.3795, 70.4291) (45.3617, 70.4402) (45.3433, 70.4517) (45.3243, 70.4621) (45.3048, 70.4714) (45.2846, 70.481) (45.2639, 70.4894) (45.2427, 70.4965) (45.221, 70.5037) (45.1989, 70.5095) (45.1765, 70.5141) (45.1606, 70.5174) (45.1446, 70.5201) (45.1285, 70.5225) (45.0513, 70.5342) (44.9734, 70.5409) (44.8962, 70.5524) (44.819, 70.5638) (44.7426, 70.58) (44.6653, 70.5912) (44.6492, 70.5935) (44.6331, 70.5957) (44.6169, 70.5971) (44.5941, 70.5992) (44.5713, 70.6001) (44.5484, 70.5994) (44.5261, 70.5988) (44.5038, 70.5968) (44.4818, 70.5935) (44.4603, 70.5902) (44.4391, 70.5858) (44.4182, 70.5801) (44.398, 70.5747) (44.3781, 70.5681) (44.3585, 70.5606) (44.3396, 70.5533) (44.3211, 70.545) (44.3031, 70.5359) (44.2855, 70.527) (44.2684, 70.5173) (44.2518, 70.5069) (44.2356, 70.4968) (44.2198, 70.4859) (44.2045, 70.4745) (44.1895, 70.4632) (44.1749, 70.4514) (44.1609, 70.4391) (44.147, 70.4269) (44.1335, 70.4143) (44.1205, 70.4011) (44.1077, 70.3881) (44.0952, 70.3747) (44.0832, 70.3609) (44.0712, 70.3471) (44.0597, 70.3329) (44.0485, 70.3184) (44.0374, 70.3039) (44.0267, 70.289) (44.0163, 70.2739) (44.0059, 70.2587) (43.9959, 70.2431) (43.9864, 70.2273) (43.9767, 70.2114) (43.9674, 70.1951) (43.9585, 70.1787) (43.9494, 70.162) (43.9408, 70.1451) (43.9325, 70.1281) (43.9241, 70.1107) (43.9161, 70.0931) (43.9085, 70.0754) (43.9007, 70.0573) (43.8933, 70.039) (43.8863, 70.0206) (43.8791, 70.0018) (43.8723, 69.9829) (43.8659, 69.9638) (43.8593, 69.9443) (43.8531, 69.9246) (43.8472, 69.9049) (43.8412, 69.8846) (43.8356, 69.8643) (43.8304, 69.8438) (43.825, 69.8229) (43.82, 69.8018) (43.8153, 69.7807) (43.8106, 69.759) (43.8062, 69.7373) (43.8021, 69.7155) (43.798, 69.6931) (43.7942, 69.6706) (43.7907, 69.6481) (43.7872, 69.6251) (43.784, 69.6019) (43.7813, 69.5787) (43.7785, 69.5549) (43.7762, 69.531) (43.7738, 69.5072) (43.7713, 69.4828) (43.7686, 69.4585) (43.7682, 69.4337) (43.7678, 69.404) (43.7707, 69.3737) (43.7645, 69.3456) (43.7564, 69.3086) (43.7323, 69.2754) (43.7119, 69.2418) (43.701, 69.2238) (43.6911, 69.2056) (43.6806, 69.1877) (43.6687, 69.1674) (43.6559, 69.1474) (43.643, 69.1276) (43.6286, 69.1055) (43.6139, 69.0836) (43.5988, 69.0619) (43.5821, 69.038) (43.565, 69.0143) (43.5475, 68.9909) (43.5283, 68.9654) (43.5087, 68.9401) (43.4887, 68.9152) (43.467, 68.8881) (43.4448, 68.8613) (43.4221, 68.835) (43.3977, 68.8065) (43.3727, 68.7785) (43.3473, 68.7508) (43.3201, 68.7212) (43.2923, 68.692) (43.264, 68.6632) (43.2338, 68.6325) (43.2031, 68.6023) (43.1719, 68.5726) (43.1386, 68.541) (43.1048, 68.51) (43.0706, 68.4795) (42.9553, 68.377) (42.8344, 68.2809) (42.7093, 68.1905) knots 0 0 0 0 0.065113 0.065113 0.065113 0.084473 0.084473 0.084473 0.102659 0.102659 0.102659 0.119672 0.119672 0.119672 0.135512 0.135512 0.135512 0.150178 0.150178 0.150178 0.163672 0.163672 0.163672 0.175991 0.175991 0.175991 0.187138 0.187138 0.187138 0.197111 0.197111 0.197111 0.205911 0.205911 0.205911 0.222284 0.222284 0.222284 0.234681 0.234681 0.234681 0.24506 0.24506 0.24506 0.255176 0.255176 0.255176 0.265035 0.265035 0.265035 0.274643 0.274643 0.274643 0.284008 0.284008 0.284008 0.293139 0.293139 0.293139 0.302047 0.302047 0.302047 0.310743 0.310743 0.310743 0.319241 0.319241 0.319241 0.327556 0.327556 0.327556 0.335706 0.335706 0.335706 0.343713 0.343713 0.343713 0.351599 0.351599 0.351599 0.359392 0.359392 0.359392 0.367126 0.367126 0.367126 0.374835 0.374835 0.374835 0.382562 0.382562 0.382562 0.390352 0.390352 0.390352 0.398256 0.398256 0.398256 0.406325 0.406325 0.406325 0.41461 0.41461 0.41461 0.423156 0.423156 0.423156 0.431994 0.431994 0.431994 0.441132 0.441132 0.441132 0.450548 0.450548 0.450548 0.460189 0.460189 0.460189 0.467051 0.467051 0.467051 0.5 0.5 0.5 0.532949 0.532949 0.532949 0.539811 0.539811 0.539811 0.549452 0.549452 0.549452 0.558868 0.558868 0.558868 0.568006 0.568006 0.568006 0.576844 0.576844 0.576844 0.58539 0.58539 0.58539 0.593675 0.593675 0.593675 0.601744 0.601744 0.601744 0.609648 0.609648 0.609648 0.617438 0.617438 0.617438 0.625165 0.625165 0.625165 0.632874 0.632874 0.632874 0.640608 0.640608 0.640608 0.648401 0.648401 0.648401 0.656287 0.656287 0.656287 0.664294 0.664294 0.664294 0.672444 0.672444 0.672444 0.680759 0.680759 0.680759 0.689257 0.689257 0.689257 0.697953 0.697953 0.697953 0.706861 0.706861 0.706861 0.715992 0.715992 0.715992 0.725357 0.725357 0.725357 0.734965 0.734965 0.734965 0.744824 0.744824 0.744824 0.75494 0.75494 0.75494 0.765319 0.765319 0.765319 0.777716 0.777716 0.777716 0.794089 0.794089 0.794089 0.802889 0.802889 0.802889 0.812862 0.812862 0.812862 0.824009 0.824009 0.824009 0.836328 0.836328 0.836328 0.849822 0.849822 0.849822 0.864488 0.864488 0.864488 0.880328 0.880328 0.880328 0.897341 0.897341 0.897341 0.915527 0.915527 0.915527 0.934887 0.934887 0.934887 1 1 1 1
  arc A280 (46.3033, 67.6574) -> (47.292, 67.7711) centre (45.7832, 76.5321) ccw
  spline S78 degree 3 poles (50.671, 69.1064) (50.5288, 69.1661) (50.3892, 69.2323) (50.2536, 69.3059) (50.2133, 69.3278) (50.1734, 69.3503) (50.1338, 69.3736) (50.0967, 69.3954) (50.0599, 69.4178) (50.0235, 69.4409) (49.9895, 69.4624) (49.9558, 69.4846) (49.9225, 69.5073) (49.8915, 69.5284) (49.8608, 69.5501) (49.8305, 69.5722) (49.8025, 69.5927) (49.7748, 69.6137) (49.7474, 69.6352) (49.7223, 69.6549) (49.6975, 69.6751) (49.673, 69.6956) (49.6507, 69.7144) (49.6286, 69.7336) (49.6069, 69.7531) (49.5873, 69.7708) (49.5681, 69.7888) (49.549, 69.8071) (49.5319, 69.8234) (49.5149, 69.84) (49.4987, 69.8571) (49.4844, 69.8721) (49.4707, 69.8876) (49.4559, 69.9026) (49.4284, 69.9307) (49.3975, 69.9575) (49.3811, 69.9918) (49.3687, 70.0177) (49.3646, 70.0479) (49.3575, 70.0767) (49.3515, 70.1008) (49.3434, 70.1238) (49.3354, 70.1471) (49.3276, 70.1697) (49.32, 70.1924) (49.3119, 70.215) (49.3039, 70.237) (49.2956, 70.2588) (49.2869, 70.2804) (49.2784, 70.3016) (49.2696, 70.3226) (49.2605, 70.3434) (49.2516, 70.3638) (49.2424, 70.3839) (49.2328, 70.404) (49.2235, 70.4235) (49.2138, 70.4428) (49.2038, 70.462) (49.1941, 70.4807) (49.184, 70.4993) (49.1736, 70.5176) (49.1634, 70.5355) (49.1529, 70.5533) (49.1421, 70.5708) (49.1315, 70.5879) (49.1205, 70.6048) (49.1093, 70.6215) (49.0982, 70.6378) (49.0869, 70.6539) (49.0752, 70.6698) (49.0637, 70.6853) (49.0519, 70.7006) (49.0398, 70.7156) (49.0279, 70.7304) (49.0156, 70.7449) (49.0031, 70.7591) (48.9907, 70.773) (48.9779, 70.7867) (48.9649, 70.8001) (48.9519, 70.8133) (48.9387, 70.8261) (48.9251, 70.8386) (48.9116, 70.851) (48.8978, 70.8631) (48.8836, 70.8747) (48.8695, 70.8863) (48.855, 70.8974) (48.8402, 70.9081) (48.8254, 70.9189) (48.8102, 70.9291) (48.7947, 70.9389) (48.7791, 70.9487) (48.7631, 70.958) (48.7468, 70.9667) (48.7303, 70.9755) (48.7135, 70.9837) (48.6963, 70.9912) (48.6788, 70.9989) (48.661, 71.0059) (48.6429, 71.0121) (48.6243, 71.0184) (48.6055, 71.024) (48.5864, 71.0286) (48.5667, 71.0334) (48.5468, 71.0373) (48.5267, 71.0401) (48.506, 71.043) (48.4851, 71.0449) (48.4642, 71.0456) (48.4425, 71.0463) (48.4208, 71.0459) (48.3992, 71.0442) (48.377, 71.0424) (48.3548, 71.0393) (48.333, 71.0348) (48.3106, 71.0303) (48.2885, 71.0242) (48.2668, 71.017) (48.2514, 71.0119) (48.2362, 71.0062) (48.221, 71.0003) (48.1483, 70.9718) (48.0775, 70.9387) (48.0049, 70.91) (47.9324, 70.8813) (47.858, 70.8571) (47.7855, 70.8282) (47.7704, 70.8222) (47.7554, 70.8159) (47.7407, 70.8091) (47.7199, 70.7996) (47.6997, 70.7888) (47.6802, 70.7769) (47.6612, 70.7652) (47.6429, 70.7523) (47.6255, 70.7384) (47.6085, 70.7249) (47.5924, 70.7104) (47.5771, 70.6951) (47.5623, 70.6802) (47.5483, 70.6646) (47.5352, 70.6483) (47.5225, 70.6325) (47.5106, 70.6161) (47.4995, 70.5991) (47.4888, 70.5827) (47.4788, 70.5657) (47.4696, 70.5484) (47.4606, 70.5315) (47.4524, 70.5142) (47.4448, 70.4967) (47.4375, 70.4795) (47.4308, 70.462) (47.4247, 70.4442) (47.4188, 70.4267) (47.4135, 70.4091) (47.4088, 70.3912) (47.4041, 70.3735) (47.4001, 70.3556) (47.3966, 70.3377) (47.3931, 70.3197) (47.3902, 70.3017) (47.3878, 70.2836) (47.3854, 70.2654) (47.3835, 70.2472) (47.3822, 70.2289) (47.3808, 70.2105) (47.3799, 70.192) (47.3795, 70.1736) (47.3791, 70.1549) (47.3791, 70.1362) (47.3796, 70.1175) (47.3802, 70.0986) (47.3811, 70.0796) (47.3825, 70.0607) (47.3839, 70.0415) (47.3858, 70.0222) (47.388, 70.0031) (47.3903, 69.9835) (47.3931, 69.964) (47.3962, 69.9445) (47.3994, 69.9246) (47.403, 69.9048) (47.4069, 69.8851) (47.411, 69.8649) (47.4154, 69.8448) (47.4202, 69.8247) (47.4252, 69.8042) (47.4305, 69.7838) (47.4362, 69.7635) (47.442, 69.7426) (47.4482, 69.7219) (47.4547, 69.7013) (47.4614, 69.6801) (47.4685, 69.6591) (47.4759, 69.6382) (47.4835, 69.6167) (47.4914, 69.5954) (47.4997, 69.5742) (47.5082, 69.5524) (47.517, 69.5308) (47.5262, 69.5093) (47.5357, 69.4873) (47.5457, 69.4655) (47.5554, 69.4437) (47.5655, 69.4212) (47.5753, 69.3988) (47.5874, 69.3772) (47.6019, 69.3513) (47.6196, 69.3265) (47.6282, 69.2991) (47.6397, 69.2629) (47.6355, 69.2222) (47.6346, 69.1829) (47.6341, 69.1618) (47.6346, 69.1411) (47.6345, 69.1204) (47.6343, 69.0968) (47.6333, 69.0732) (47.632, 69.0495) (47.6306, 69.0231) (47.6288, 68.9968) (47.6266, 68.9705) (47.6241, 68.9414) (47.6211, 68.9124) (47.6176, 68.8834) (47.6138, 68.8517) (47.6095, 68.82) (47.6046, 68.7884) (47.5994, 68.7541) (47.5935, 68.7198) (47.5871, 68.6857) (47.5801, 68.6488) (47.5725, 68.612) (47.5643, 68.5754) (47.5556, 68.5361) (47.5461, 68.4969) (47.536, 68.4579) (47.5252, 68.4162) (47.5137, 68.3746) (47.5015, 68.3333) (47.4885, 68.2893) (47.4748, 68.2456) (47.4603, 68.202) (47.4117, 68.0556) (47.3551, 67.9119) (47.292, 67.7711) knots 0 0 0 0 0.065113 0.065113 0.065113 0.084473 0.084473 0.084473 0.102659 0.102659 0.102659 0.119672 0.119672 0.119672 0.135512 0.135512 0.135512 0.150178 0.150178 0.150178 0.163672 0.163672 0.163672 0.175991 0.175991 0.175991 0.187138 0.187138 0.187138 0.197111 0.197111 0.197111 0.205911 0.205911 0.205911 0.222284 0.222284 0.222284 0.234681 0.234681 0.234681 0.24506 0.24506 0.24506 0.255176 0.255176 0.255176 0.265035 0.265035 0.265035 0.274643 0.274643 0.274643 0.284008 0.284008 0.284008 0.293139 0.293139 0.293139 0.302047 0.302047 0.302047 0.310743 0.310743 0.310743 0.319241 0.319241 0.319241 0.327556 0.327556 0.327556 0.335706 0.335706 0.335706 0.343713 0.343713 0.343713 0.351599 0.351599 0.351599 0.359392 0.359392 0.359392 0.367126 0.367126 0.367126 0.374835 0.374835 0.374835 0.382562 0.382562 0.382562 0.390352 0.390352 0.390352 0.398256 0.398256 0.398256 0.406325 0.406325 0.406325 0.41461 0.41461 0.41461 0.423156 0.423156 0.423156 0.431994 0.431994 0.431994 0.441132 0.441132 0.441132 0.450548 0.450548 0.450548 0.460189 0.460189 0.460189 0.467051 0.467051 0.467051 0.5 0.5 0.5 0.532949 0.532949 0.532949 0.539811 0.539811 0.539811 0.549452 0.549452 0.549452 0.558868 0.558868 0.558868 0.568006 0.568006 0.568006 0.576844 0.576844 0.576844 0.58539 0.58539 0.58539 0.593675 0.593675 0.593675 0.601744 0.601744 0.601744 0.609648 0.609648 0.609648 0.617438 0.617438 0.617438 0.625165 0.625165 0.625165 0.632874 0.632874 0.632874 0.640608 0.640608 0.640608 0.648401 0.648401 0.648401 0.656287 0.656287 0.656287 0.664294 0.664294 0.664294 0.672444 0.672444 0.672444 0.680759 0.680759 0.680759 0.689257 0.689257 0.689257 0.697953 0.697953 0.697953 0.706861 0.706861 0.706861 0.715992 0.715992 0.715992 0.725357 0.725357 0.725357 0.734965 0.734965 0.734965 0.744824 0.744824 0.744824 0.75494 0.75494 0.75494 0.765319 0.765319 0.765319 0.777716 0.777716 0.777716 0.794089 0.794089 0.794089 0.802889 0.802889 0.802889 0.812862 0.812862 0.812862 0.824009 0.824009 0.824009 0.836328 0.836328 0.836328 0.849822 0.849822 0.849822 0.864488 0.864488 0.864488 0.880328 0.880328 0.880328 0.897341 0.897341 0.897341 0.915527 0.915527 0.915527 0.934887 0.934887 0.934887 1 1 1 1
  arc A281 (50.671, 69.1064) -> (51.4704, 69.6993) centre (45.7832, 76.5321) ccw